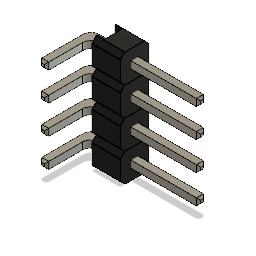
pinsBentMale (Autodesk Fusion 360 design; units mm, degrees)
Autodesk Fusion 360 part; units mm, degrees
note: some values were not read from the file. Set by a fixed rule: which sketch regions a step uses.
sketch "Sketch1" plane through (0, 0, 0) normal (0, 1, 0) x (1, 0, 0) in component "Pin"
  line L0 (11.684, 0) -> (11.684, -0.635)
  line L1 (0, -0.3175) -> (1.524, -0.3175) construction
  line L2 (1.524, 0) -> (1.524, -4.572)
  line L3 (1.524, 0) -> (11.684, 0)
  line L4 (11.684, -0.635) -> (2.159, -0.635)
  line L5 (2.159, -0.635) -> (1.524, -0.635) construction
  line L6 (2.159, -0.635) -> (2.159, -4.572)
  line L7 (2.159, -4.572) -> (1.524, -4.572)
  dimension "d3" = 11.684
  dimension "d19" = 1.524
  dimension "d20" = 0.635
  dimension "d21" = 4.572
  measures "d3" distance of origin
  measures "d19" distance of origin
extrude "Extrude1" add sketch "Sketch1" along normal blind 0.635 makes body 1 in component "Pin"
fillet "Fillet1" radius 0.75 2 edges at (2.159, 0.3175, 0.635) (1.524, 0.3175, 0) on bodies 1 in component "Pin"
chamfer "Chamfer1" distance 0.1905 angle 45 8 edges at (11.684, 0.3175, 0.635) (11.684, 0.635, 0.3175) (11.684, 0.3175, 0) (11.684, 0, 0.3175) (2.159, 0.3175, 4.572) (1.524, 0.3175, 4.572) (1.8415, 0.635, 4.572) (1.8415, 0, 4.572) on bodies 1 in component "Pin"
sketch "Sketch1 (2)" plane through (0, 0, 0) normal (0, 0, 1) x (1, 0, 0)
  line L0 (0, 0.3175) -> (0, 14)
  line L1 (1.7145, 0.1905) -> (1.7145, 0.4445)
  line L2 (1.7145, 0.3175) -> (0, 0.3175) construction
sketch "Sketch1 (3)" plane through (0, 0, 0) normal (0, 1, 0) x (1, 0, 0) in component "Plastic"
  line L0 (0, -0.3175) -> (3.81, -0.3175)
  line L1 (3.81, -1.0795) -> (3.81, 0.4445)
  line L2 (3.81, 0.4445) -> (3.81, 0.9525) construction
  line L3 (3.81, -1.0795) -> (3.81, -1.5875) construction
  line L4 (3.81, 0.4445) -> (3.175, 0.4445)
  line L5 (3.81, -1.0795) -> (3.175, -1.0795)
  line L6 (3.175, -1.0795) -> (3.175, -1.5875)
  line L7 (3.175, 0.4445) -> (3.175, 0.9525)
  line L8 (3.175, 0.9525) -> (5.715, 0.9525)
  line L9 (5.715, 0.9525) -> (5.715, -1.5875)
  line L10 (3.175, -1.5875) -> (5.715, -1.5875)
  dimension "d7" = 3.81
  dimension "d8" = 1.524
  dimension "d9" = 0.508
  dimension "d11" = 0.635
  dimension "d12" = 2.54
  measures "d7" distance of origin
extrude "Extrude1'" add sketch "Sketch1 (3)" along normal mid plane 2.54 from surface at 0.3175 separate body makes body 2 in component "Plastic"
chamfer "Chamfer1'" distance 0.4 angle 45 4 edges at (4.445, 1.5875, -0.9525) (4.445, -0.9525, -0.9525) (4.445, 1.5875, 1.5875) (4.445, -0.9525, 1.5875) on bodies 2 in component "Plastic"
other "PathPattern2"
component "Header" placed x (1, 0, 0) y (0, 1, 0) z (0, 0, 1) at (0, 0, 0)
component "Header" placed x (1, 0, 0) y (0, 1, 0) z (0, 0, 1) at (0, 2.54, 0)
component "Header" placed x (1, 0, 0) y (0, 1, 0) z (0, 0, 1) at (0, 5.08, 0)
component "Header" placed x (1, 0, 0) y (0, 1, 0) z (0, 0, 1) at (0, 7.62, 0)
component "Pin" placed x (1, 0, 0) y (0, 1, 0) z (0, 0, 1) at (0, 0, 0) in component "Header"
component "Plastic" placed x (1, 0, 0) y (0, 1, 0) z (0, 0, 1) at (0, 0, 0) in component "Header"
equation "pinCount = 4"
equation "d13 = 0.025 in / 2"
equation "d23 = pinCount"
